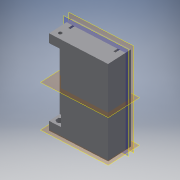
# Autodesk Inventor part: Caixa Painel
Saved by Autodesk Inventor 2019 (Build 230136000, 136)
## iProperties
Created: 2020-05-29
Part Number: Caixa Painel
Material: Generic
Document SubType Name: Modeling
Designer: luiza
Density: 1 g/cm^3
Appearance: Default
Categories: <MemberInstance><Categories><Category DisplayName="" Mnemonic="CABLEANDHARNESS" InternalName="e4a7e005-5e42-4d16-b293-125e7f0d0512"><Category DisplayName="" Mnemonic="CONNECTORS" InternalName="6f634eba-a678-4820-a31d-2c2d5ee6728e"><CategoryParameter DisplayName="" Mnemonic="REFDES" InternalName="c3740e8c-60ab-4d5d-8584-52b73222f2f0"/><Category DisplayName="" Mnemonic="DISCRETEWIRE" InternalName="9a3407de-09b2-4cdb-8c40-9708d5144a28"/></Category></Category></Categories><FamilyTemplate><FamilyTemplateParameters></FamilyTemplateParameters></FamilyTemplate><CategoryParameterMap><ParamToTemplateMap><ParamToTemplate CategoryParameter="//CategoryParameter[@InternalName='c3740e8c-60ab-4d5d-8584-52b73222f2f0']" ConstantValue=""/></ParamToTemplateMap></CategoryParameterMap></MemberInstance>
Author: luiza
Autodesk Inventor part; units mm, degrees
ref_plane "YZ Plane" through (0, 0, 0) normal (1, 0, 0) x (0, 1, 0)
ref_plane "XZ Plane" through (0, 0, 0) normal (0, 1, 0) x (-1, 0, 0)
ref_plane "XY Plane" through (0, 0, 0) normal (0, 0, 1) x (1, 0, 0)
ref_plane "Work Plane1" through (-1405.2046, 1188.2554, 32.7938) normal (0.0525168, 0, 0.99862) x (0, -1, 0)
sketch "Sketch1" plane through (-1405.2046, 1188.2554, 32.7938) normal (0.0525168, 0, 0.99862) x (0, -1, 0)
  line L0 (-58, 47) -> (58, 47)
  line L1 (72, 33) -> (72, -33)
  line L2 (58, -47) -> (-58, -47)
  line L3 (-72, -33) -> (-72, 33)
  line L4 (-65, 33) -> (-72, 33)
  line L5 (-58, 40) -> (-58, 47)
  arc A0 (-65, 33) -> (-58, 40) centre (-65, 40) ccw
  line L6 (0, 69.334) -> (0, -92.7299)
  line L7 (101.325, 0) -> (-113.3608, 0)
  line L8 (65, 33) -> (72, 33)
  line L9 (58, 40) -> (58, 47)
  arc A1 (58, 40) -> (65, 33) centre (65, 40) ccw
  line L10 (-65, -33) -> (-72, -33)
  line L11 (-58, -40) -> (-58, -47)
  arc A2 (-58, -40) -> (-65, -33) centre (-65, -40) ccw
  line L12 (58, -40) -> (58, -47)
  arc A3 (65, -33) -> (58, -40) centre (65, -40) ccw
  line L13 (65, -33) -> (72, -33)
  line L14 (75, -50) -> (75, 50)
  line L15 (75, 50) -> (-75, 50)
  line L16 (-75, 50) -> (-75, -50)
  line L17 (-75, -50) -> (75, -50)
  constraints: 36 end point, 15 symmetric about line, 8 point on circle, 4 centre point, 4 horizontal, 4 vertical, 1 coincident, 7 other
extrude "Extrusion1" add sketch "Sketch1" along normal blind 40 contours L5 A0 L4 L3 L7 L16 L15 L6 L0 | L6 L15 L14 L7 L1 L8 A1 L9 L0 | L6 L17 L16 L7 L3 L10 A2 L11 L2 | L2 L12 A3 L13 L1 L7 L14 L17 L6
sketch "Sketch2" plane through (-1403.1039, 1188.2554, 72.7386) normal (0.0525168, 0, 0.99862) x (0, -1, 0)
  line L0 (72, -33) -> (65, -33) projected
  arc A0 (65, -33) -> (58, -40) centre (65, -40) ccw projected
  line L1 (58, -40) -> (58, -47) projected
  line L2 (58, -47) -> (-58, -47) projected
  line L3 (-58, -47) -> (-58, -40) projected
  arc A1 (-58, -40) -> (-65, -33) centre (-65, -40) ccw projected
  line L4 (-65, -33) -> (-72, -33) projected
  line L5 (-72, -33) -> (-72, 33) projected
  line L6 (-72, 33) -> (-65, 33) projected
  arc A2 (-65, 33) -> (-58, 40) centre (-65, 40) ccw projected
  line L7 (-58, 40) -> (-58, 47) projected
  line L8 (-58, 47) -> (58, 47) projected
  line L9 (58, 47) -> (58, 40) projected
  arc A3 (58, 40) -> (65, 33) centre (65, 40) ccw projected
  line L10 (65, 33) -> (72, 33) projected
  line L11 (72, 33) -> (72, -33) projected
  line L12 (-75, 50) -> (75, 50)
  line L13 (75, 50) -> (75, -50)
  line L14 (75, -50) -> (-75, -50)
  line L15 (-75, -50) -> (-75, 50)
  point P0 (75, -40)
  constraints: 8 end point, 2 horizontal, 2 vertical, 4 other
extrude "Extrusion2" add sketch "Sketch2" along normal blind 3 contours L0 A0 L1 L2 L3 A1 L4 L5 L6 A2 L7 L8 L9 A3 L10 L11 | L12 L13 L14 L15
ref_plane "Work Plane2" through (-1404.6794, 1188.2554, 42.78) normal (-0.0525168, 0, -0.99862) x (0, -1, 0)
sketch "Sketch3" plane through (-1404.6794, 1188.2554, 42.78) normal (-0.0525168, 0, -0.99862) x (0, -1, 0)
  line L0 (72, -33) -> (72, 33) projected
  line L1 (72, 0) -> (-85.4188, 0)
  line L2 (0, -47) -> (0, 56.7085)
  line L3 (-60.8962, 40.0088) -> (-77.9922, 40.0088)
  line L4 (-64.8068, 40.0088) -> (-83.3652, 40.0088) construction
  arc A0 (-65, 33) -> (-58, 40) centre (-65, 40) ccw projected
  line L5 (-65, 33) -> (-65, 47.1957)
  line L6 (-62.9449, 36.4573) -> (-67.0449, 36.4573)
  line L7 (-67.0449, 36.4573) -> (-69.0936, 40.0088)
  line L8 (-69.0936, 40.0088) -> (-67.0449, 43.5602)
  line L9 (-67.0449, 43.5602) -> (-62.9449, 43.5602)
  line L10 (-62.9449, 43.5602) -> (-60.8962, 40.0088)
  line L11 (-60.8962, 40.0088) -> (-62.9449, 36.4573)
  line L12 (62.9449, 36.4573) -> (67.0449, 36.4573)
  line L13 (67.0449, 36.4573) -> (69.0936, 40.0088)
  line L14 (69.0936, 40.0088) -> (67.0449, 43.5602)
  line L15 (67.0449, 43.5602) -> (62.9449, 43.5602)
  line L16 (62.9449, 43.5602) -> (60.8962, 40.0088)
  line L17 (60.8962, 40.0088) -> (62.9449, 36.4573)
  line L18 (-62.9449, -36.4573) -> (-67.0449, -36.4573)
  line L19 (-67.0449, -36.4573) -> (-69.0936, -40.0088)
  line L20 (-69.0936, -40.0088) -> (-67.0449, -43.5602)
  line L21 (-67.0449, -43.5602) -> (-62.9449, -43.5602)
  line L22 (-62.9449, -43.5602) -> (-60.8962, -40.0088)
  line L23 (-60.8962, -40.0088) -> (-62.9449, -36.4573)
  line L24 (62.9449, -43.5602) -> (60.8962, -40.0088)
  line L25 (60.8962, -40.0088) -> (62.9449, -36.4573)
  line L26 (62.9449, -36.4573) -> (67.0449, -36.4573)
  line L27 (67.0449, -43.5602) -> (62.9449, -43.5602)
  line L28 (69.0936, -40.0088) -> (67.0449, -43.5602)
  line L29 (67.0449, -36.4573) -> (69.0936, -40.0088)
  point P0 (1188.2554, -1404.9877)
  point P1 (64.8068, 40.0088)
  point P2 (65, 40)
  point P3 (-64.8068, -40.0088)
  point P4 (-65, -40)
  point P5 (64.8068, -40.0088)
  point P6 (65, -40)
  dimension "d114" = 4.1
  dimension "d115" = 7.1029
  constraints: 58 end point, 24 symmetric about line, 5 equal length, 5 horizontal, 2 vertical, 1 collinear, 1 midpoint, 1 parallel, 1 point on line
  measures "d114" distance of L3.start L6.start
  measures "d115" distance of L8.end L6.end
extrude "Extrusion5" cut sketch "Sketch3" against normal blind 5.1
sketch "Sketch4" plane through (-1405.2046, 1188.2554, 32.7938) normal (-0.0525168, 0, -0.99862) x (0, -1, 0)
  line L0 (65, 33) -> (72, 33) projected
  line L1 (72, 33) -> (72, -33) projected
  line L2 (72, -33) -> (65, -33) projected
  arc A0 (65, -33) -> (58, -40) centre (65, -40) ccw projected
  line L3 (58, -40) -> (58, -47) projected
  line L4 (58, -47) -> (-58, -47) projected
  line L5 (-58, -47) -> (-58, -40) projected
  arc A1 (-58, -40) -> (-65, -33) centre (-65, -40) ccw projected
  line L6 (-65, -33) -> (-72, -33) projected
  line L7 (-72, -33) -> (-72, 33) projected
  line L8 (-72, 33) -> (-65, 33) projected
  arc A2 (-65, 33) -> (-58, 40) centre (-65, 40) ccw projected
  line L9 (-58, 40) -> (-58, 47) projected
  line L10 (-58, 47) -> (58, 47) projected
  line L11 (58, 47) -> (58, 40) projected
  arc A3 (58, 40) -> (65, 33) centre (65, 40) ccw projected
  circle A4 centre (-65, 40) radius 2
  circle A5 centre (65, 40) radius 2
  circle A6 centre (65, -40) radius 2
  circle A7 centre (-65, -40) radius 2
  point P0 (1188.2554, -1404.9877)
  dimension "d19" = 4
  dimension "d20" = 4
  dimension "d21" = 4
  dimension "d22" = 4
  constraints: 4 centre point
  measures "d19" diameter of A7
  measures "d20" diameter of A4
  measures "d21" diameter of A5
  measures "d22" diameter of A6
extrude "Extrusion6" cut sketch "Sketch4" against normal blind 24 contours A4 | A5 | A6 | A7
sketch "Sketch15" plane through (-1455.1356, 1113.2554, 35.4196) normal (0, -1, 0) x (0.99862, 0, -0.0525168)
  circle A0 centre (10, 33) radius 3
  line L0 (0, 40) -> (100, 40) projected
  line L1 (0, 0) -> (0, 40) projected
  point P0 (1454.9877, 41.0484)
  dimension "d74" = 7
  dimension "d75" = 6
  dimension "d76" = 10
  constraints: 1 centre point
  measures "d74" distance from line of L0 A0.centre
  measures "d75" diameter of A0
  measures "d76" distance from line of L1 A0.centre
extrude "Extrusion14" cut sketch "Sketch15" against normal through all
ref_plane "Work Plane7" through (-1438.1591, 1114.7554, 34.5268) normal (0, 1, 0) x (0.99862, 0, -0.0525168)
sketch "Sketch16" plane through (-1438.1591, 1114.7554, 34.5268) normal (0, 1, 0) x (0.99862, 0, -0.0525168)
  line L0 (-17, 0) -> (-17, -43) projected
  line L1 (-17, -43) -> (3, -43)
  line L2 (3, -43) -> (3, -23)
  line L3 (3, -23) -> (-17, -23)
  line L4 (-17, -23) -> (-17, -43)
  circle A0 centre (-7, -33) radius 3 projected
  dimension "d79" = 10
  dimension "d80" = 10
  constraints: 8 end point, 2 parallel, 1 horizontal, 1 perpendicular
  measures "d79" distance from line of L2 A0.centre
  measures "d80" distance from line of L3 A0.centre
extrude "Extrusion15" cut sketch "Sketch16" along normal up to surface (145.5 mm away)
sketch "Sketch17" plane through (-1438.1591, 1260.2554, 34.5268) normal (0, -1, 0) x (0.99862, 0, -0.0525168)
  line L0 (-17, 43) -> (3, 43) projected
  line L1 (-17, 23) -> (-17, 43) projected
  line L2 (-7, 23) -> (-14, 23) projected
  line L3 (3, 40) -> (3, 43) projected
  line L4 (3, 43) -> (3, 23)
  line L5 (-17, 23) -> (3, 23)
  line L6 (8, 18) -> (-17, 18)
  line L7 (8, 43) -> (8, 18)
  line L8 (83, 43) -> (-17, 43) projected
  line L9 (8, 43) -> (3, 43)
  line L10 (-17, 23) -> (-17, 18)
  line L11 (-17, 0) -> (-17, 43) projected
  dimension "d83" = 5
  constraints: 12 end point, 2 point on line, 1 collinear, 1 horizontal, 1 vertical
  measures "d83" distance between parallel lines of L4 L7
extrude "Extrusion16" add sketch "Sketch17" along normal up to surface (144 mm away) contours L8 L7 L6 L10 L5 L2 L4 L3
sketch "Sketch18" plane through (-1433.9553, 1260.2554, 57.3375) normal (0, -1, 0) x (0.99862, 0, -0.0525168)
  circle A0 centre (-10, 10) radius 3 projected
  circle A1 centre (-10, 10) radius 6.3509 construction
  line L0 (-10, 16.3509) -> (-4.5, 13.1754)
  line L1 (-4.5, 13.1754) -> (-4.5, 6.8246)
  line L2 (-4.5, 6.8246) -> (-10, 3.6491)
  line L3 (-10, 3.6491) -> (-15.5, 6.8246)
  line L4 (-15.5, 6.8246) -> (-15.5, 13.1754)
  line L5 (-15.5, 13.1754) -> (-10, 16.3509)
  line L6 (-15.5, 10) -> (-4.5, 10)
  line L7 (0, 0) -> (0, 20) projected
  line L8 (-20, 20) -> (0, 20) projected
  line L9 (-20, 0) -> (-20, 20) projected
  line L10 (-20, 0) -> (0, 0) projected
  circle A2 centre (-10, 10) radius 3 projected
  dimension "d89" = 11
  constraints: 14 end point, 6 point on circle, 3 equal length, 2 midpoint, 2 vertical, 1 centre point, 1 coincident, 1 parallel
  measures "d89" distance of L6.start L6.end
extrude "Extrusion17" add sketch "Sketch18" along normal blind 10
ref_plane "Work Plane8" through (-1455.1356, 1188.2554, 35.4196) normal (0, 1, 0) x (0.99862, 0, -0.0525168)
mirror "Mirror4" about plane through (-1455.1356, 1188.2554, 35.4196) normal (0, 1, 0) of "Extrusion17"
sketch "Sketch19" plane through (-1438.1591, 1114.7554, 34.5268) normal (0, 1, 0) x (0.99862, 0, -0.0525168)
  circle A0 centre (-7, -33) radius 3 projected
  line L0 (3, -43) -> (-17, -43) projected
  line L1 (3, -43) -> (3, -23) projected
  line L2 (3, -23) -> (-17, -23) projected
  line L3 (-17, -43) -> (-17, -23) projected
  point P0 (1437.9877, -41.0484)
extrude "Extrusion18" add sketch "Sketch19" along normal up to surface (1.5 mm away)
sketch "Sketch20" plane through (-1433.9553, 1126.2554, 57.3375) normal (0.0525168, 0, 0.99862) x (0.99862, 0, -0.0525168)
  arc A0 (-3.75, 54.75) -> (-13.25, 54.75) centre (-8.5, 54.75) ccw
  arc A1 (-13.25, 42.492) -> (-3.75, 42.492) centre (-8.5, 42.492) ccw
  line L0 (-3.75, 54.75) -> (-3.75, 42.492)
  line L1 (-13.25, 54.75) -> (-13.25, 42.492)
  line L2 (-20, 0) -> (0, 0) projected
  line L3 (0, 0) -> (0, 124) projected
  line L4 (0, 124) -> (-20, 124) projected
  line L5 (-20, 0) -> (-20, 124) projected
  line L6 (-20, 62) -> (0, 62)
  line L7 (-8.5, 124) -> (-8.5, 0)
  line L8 (-3.75, 48.621) -> (-13.25, 48.621)
  line L9 (-8.5, 59.5) -> (-8.5, 37.742)
  arc A2 (-3.75, 81.508) -> (-13.25, 81.508) centre (-8.5, 81.508) ccw
  arc A3 (-13.25, 69.25) -> (-3.75, 69.25) centre (-8.5, 69.25) ccw
  line L10 (-3.75, 81.508) -> (-3.75, 69.25)
  line L11 (-13.25, 81.508) -> (-13.25, 69.25)
  line L12 (-3.75, 75.379) -> (-13.25, 75.379)
  line L13 (-8.5, 86.258) -> (-8.5, 64.5)
  arc A4 (-3.75, 27.992) -> (-13.25, 27.992) centre (-8.5, 27.992) ccw
  arc A5 (-13.25, 15.734) -> (-3.75, 15.734) centre (-8.5, 15.734) ccw
  line L14 (-3.75, 27.992) -> (-3.75, 15.734)
  line L15 (-13.25, 27.992) -> (-13.25, 15.734)
  line L16 (-3.75, 21.863) -> (-13.25, 21.863)
  line L17 (-8.5, 32.742) -> (-8.5, 10.984)
  arc A6 (-3.75, 108.266) -> (-13.25, 108.266) centre (-8.5, 108.266) ccw
  line L18 (-3.75, 102.137) -> (-13.25, 102.137)
  line L19 (-3.75, 108.266) -> (-3.75, 96.008)
  line L20 (-13.25, 108.266) -> (-13.25, 96.008)
  line L21 (-8.5, 113.016) -> (-8.5, 91.258)
  arc A7 (-13.25, 96.008) -> (-3.75, 96.008) centre (-8.5, 96.008) ccw
  line L22 (-8.5, 62) -> (-2.9138, 62)
  line L23 (-5.7069, 62) -> (-5.7069, 75.379)
  line L24 (-5.7069, 62) -> (-5.7069, 48.621)
  point P0 (-20, 0)
  point P1 (-17, 120)
  point P2 (-8.5, 48.621)
  point P3 (-8.5, 75.379)
  point P4 (-8.5, 21.863)
  point P5 (-8.5, 102.137)
  dimension "d96" = 4.75
  dimension "d97" = 12.258
  dimension "d100" = 4.75
  dimension "d101" = 12.258
  dimension "d102" = 4.75
  dimension "d103" = 12.258
  dimension "d104" = 14.5
  dimension "d105" = 14.5
  dimension "d108" = 4.75
  dimension "d109" = 12.258
  dimension "d110" = 14.5
  dimension "d111" = 0
  constraints: 42 end point, 24 point on circle, 16 midpoint, 12 tangent, 9 vertical, 8 centre point, 5 equal length, 4 point on line, 3 perpendicular, 1 other
  measures "d96" radius of A1
  measures "d97" distance of L1.start L1.end
  measures "d100" radius of A3
  measures "d101" distance of L11.start L11.end
  measures "d102" radius of A5
  measures "d103" distance of L15.start L15.end
  measures "d104" distance of A3.centre A0.centre
  measures "d105" distance of A4.centre A1.centre
  measures "d108" radius of A7
  measures "d109" distance of L20.start L20.end
  measures "d110" distance of A7.centre A2.centre
  measures "d111" distance between parallel lines of L6 L22
extrude "Extrusion19" cut sketch "Sketch20" against normal up to next contours L7 L8 L1 A0 | A0 L24 L8 L7 | A0 L0 L8 L24 | L8 L0 A1 L7 | L7 A1 L1 L8 | A3 L11 L12 L7 | L7 L12 L23 A3 | L23 L12 L10 A3 | L12 L11 A2 L7 | L7 A2 L10 L12 | A4 L14 L16 L7 | L7 L16 L15 A4 | L16 L14 A5 L7 | L7 A5 L15 L16 | A6 L19 L18 L7 | L7 L18 L20 A6 | A7 L20 L18 L7 | L7 L18 L19 A7
body "Solid1"
